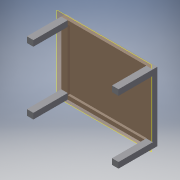
# Autodesk Inventor part: Каркас для плат
Saved by Autodesk Inventor 2019 (Build 230136000, 136)
## iProperties
Created: 2020-05-13
Part Number: Каркас для плат
Material: Типовые
Document SubType Name: Modeling
Designer: Surflay
Density: 1 g/cm^3
Appearance: По умолчанию
Author: Surflay
Autodesk Inventor part; units mm, degrees
ref_plane "YZ Plane" through (0, 0, 0) normal (1, 0, 0) x (0, 1, 0)
ref_plane "XZ Plane" through (0, 0, 0) normal (0, 1, 0) x (-1, 0, 0)
ref_plane "XY Plane" through (0, 0, 0) normal (0, 0, 1) x (1, 0, 0)
sketch "Эскиз1" plane through (0, 0, 0) normal (0, 0, 1) x (1, 0, 0)
  line L0 (0, 0) -> (80, 0)
  line L1 (80, 0) -> (80, 60)
  line L2 (80, 60) -> (0, 60)
  line L3 (0, 60) -> (0, 0)
  dimension "d0" = 60
  dimension "d1" = 80
  constraints: 8 end point, 2 parallel, 1 horizontal, 1 perpendicular
  measures "d0" distance between parallel lines of L0 L2
  measures "d1" distance between parallel lines of L1 L3
extrude "Выдавливание1" add sketch "Эскиз1" along normal blind 4
ref_plane "РабПлоскость1" through (0, 0, 4) normal (0, 0, 1) x (1, 0, 0)
sketch "Эскиз3" plane through (0, 0, 4) normal (0, 0, 1) x (1, 0, 0)
  line L0 (5.5, 56.67) -> (74.5, 56.67)
  line L1 (74.5, 56.67) -> (74.5, 3.33)
  line L2 (74.5, 3.33) -> (5.5, 3.33)
  line L3 (5.5, 3.33) -> (5.5, 56.67)
  line L4 (80, 60) -> (0, 60) projected
  line L5 (80, 0) -> (80, 60) projected
  line L6 (0, 0) -> (80, 0) projected
  dimension "d5" = 69
  dimension "d6" = 53.34
  dimension "d7" = 3.33
  dimension "d8" = 5.5
  dimension "d11" = 60
  dimension "d12" = 80
  constraints: 8 end point, 2 parallel, 1 horizontal, 1 perpendicular
  measures "d5" distance of L1.end L2.end
  measures "d6" distance between parallel lines of L2 L0
  measures "d7" distance between parallel lines of L0 L4
  measures "d8" distance between parallel lines of L1 L5
  measures "d11" distance between parallel lines of L6 L4
  measures "d12" distance of L4.start L4.end
extrude "Выдавливание2" cut sketch "Эскиз3" against normal blind 2
sketch "Эскиз4" plane through (0, 0, 4) normal (0, 0, 1) x (1, 0, 0)
  line L0 (80, 60) -> (0, 60) projected
  line L1 (0, 60) -> (0, 0) projected
  line L2 (5.5, 56.67) -> (74.5, 56.67) projected
  line L3 (5.5, 3.33) -> (5.5, 56.67) projected
  line L4 (80, 0) -> (80, 60) projected
  line L5 (74.5, 56.67) -> (74.5, 3.33) projected
  line L6 (74.5, 3.33) -> (5.5, 3.33) projected
  line L7 (0, 0) -> (80, 0) projected
  line L8 (5.5, 3.33) -> (5.5, 56.67) projected
  line L9 (0, 60) -> (5.5, 60)
  line L10 (5.5, 60) -> (5.5, 55)
  line L11 (5.5, 55) -> (0, 55)
  line L12 (0, 55) -> (0, 60)
  line L13 (80, 60) -> (0, 60) projected
  line L14 (74.5, 56.67) -> (74.5, 3.33) projected
  line L15 (80, 60) -> (74.5, 60)
  line L16 (74.5, 60) -> (74.5, 55)
  line L17 (74.5, 55) -> (80, 55)
  line L18 (80, 55) -> (80, 60)
  line L19 (80, 0) -> (74.5, 0)
  line L20 (74.5, 0) -> (74.5, 5)
  line L21 (74.5, 5) -> (80, 5)
  line L22 (80, 5) -> (80, 0)
  line L23 (0, 0) -> (5.5, 0)
  line L24 (5.5, 0) -> (5.5, 5)
  line L25 (5.5, 5) -> (0, 5)
  line L26 (0, 5) -> (0, 0)
  dimension "d13" = 5
  dimension "d14" = 5
  dimension "d15" = 5
  constraints: 32 end point, 8 parallel, 5 point on line, 4 horizontal, 4 perpendicular
  measures "d13" distance of L9.end L10.end
  measures "d14" distance of L19.end L20.end
  measures "d15" distance of L24.end L23.end
extrude "Выдавливание3" add sketch "Эскиз4" along normal blind 30 contours L4 L17 L5 L16 L0 | L10 L3 L11 L1 L0 | L4 L7 L20 L5 L21 | L25 L3 L24 L7 L1
equation "\"d7\" = -0.5 * d6 + 0.5 * d11"
equation "\"d8\" = -0.5 * d5 + 0.5 * d12"
